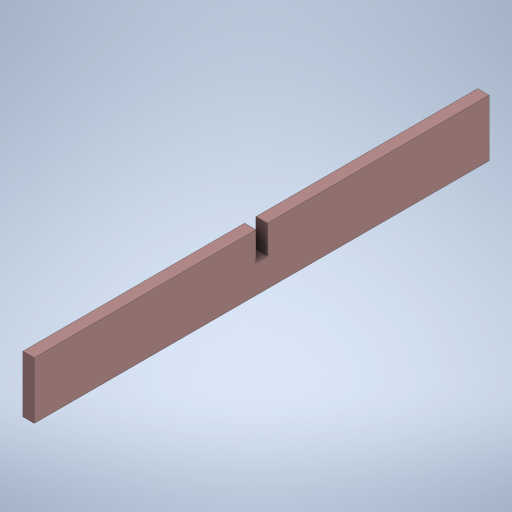
# Autodesk Inventor part: PotStand
Saved by Autodesk Inventor 2024.3 (Build 283343000, 343)
## iProperties
Created: 2025-03-01
Part Number: PotStand
Material: Generic
Document SubType Name: Modeling
Designer: ajclo
Density: 1 g/cm^3
Appearance: Default
Author: ajclo
Autodesk Inventor part; units mm, degrees
ref_plane "YZ Plane" through (0, 0, 0) normal (1, 0, 0) x (0, 1, 0)
ref_plane "XZ Plane" through (0, 0, 0) normal (0, 1, 0) x (-1, 0, 0)
ref_plane "XY Plane" through (0, 0, 0) normal (0, 0, 1) x (1, 0, 0)
sketch "Sketch1" plane through (0, 0, 0) normal (1, 0, 0) x (0, 1, 0)
  line L0 (-12.5, 100) -> (12.5, 100)
  line L1 (12.5, 100) -> (12.5, -100)
  line L2 (12.5, -100) -> (-12.5, -100)
  line L3 (-12.5, -100) -> (-12.5, 100)
  line L4 (-12.5, 100) -> (12.5, -100) construction
  line L5 (12.5, 100) -> (-12.5, -100) construction
  point P0 (0, 0)
  dimension "d0" = 200
  dimension "d1" = 25
  constraints: 12 end point, 2 midpoint, 2 parallel, 1 horizontal, 1 perpendicular
  measures "d0" distance of L0.end L1.end
  measures "d1" distance of L1.end L2.end
extrude "Extrusion1" add sketch "Sketch1" along normal blind 5
sketch "Sketch2" plane through (5, 0, 0) normal (1, 0, 0) x (0, 0, -1)
  line L0 (100, 12.5) -> (-100, 12.5) projected
  line L1 (-2.5, -12.5) -> (2.5, -12.5)
  line L2 (2.5, -12.5) -> (2.5, 12.5)
  line L3 (2.5, 12.5) -> (-2.5, 12.5)
  line L4 (-2.5, 12.5) -> (-2.5, -12.5)
  line L5 (-2.5, -12.5) -> (2.5, 12.5) construction
  line L6 (2.5, -12.5) -> (-2.5, 12.5) construction
  line L7 (-2.5, 0) -> (2.5, 0)
  point P0 (0, 0)
  dimension "d4" = 5
  constraints: 14 end point, 4 midpoint, 2 parallel, 1 horizontal, 1 perpendicular, 1 point on line
  measures "d4" distance between parallel lines of L2 L4
extrude "Extrusion2" cut sketch "Sketch2" against normal blind 5 contours L2 L7 L4 L0
body "Solid1"
